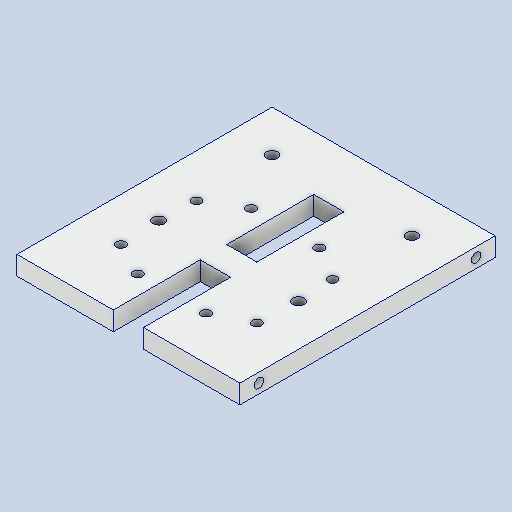
# Autodesk Inventor part: belt_liner_v2_Plate_4
Saved by Autodesk Inventor 2025.2 (Build 292293000, 293)
## iProperties
Created: 2025-01-05
Part Number: belt_liner_v2_Plate_4
Material: アルミニウム 6061
Document SubType Name: Modeling
Designer: haruy
Density: 2.7 g/cm^3
Appearance: アルミニウム - フラット
Author: haruy
Autodesk Inventor part; units mm, degrees
ref_plane "YZ Plane" through (0, 0, 0) normal (1, 0, 0) x (0, 1, 0)
ref_plane "XZ Plane" through (0, 0, 0) normal (0, 1, 0) x (-1, 0, 0)
derived "belt_liner_v2_Sketch_Base.ipt"
sketch "スケッチ4" plane through (0, 300, 0) normal (0, 1, 0) x (-1, 0, 0)
  line L0 (0, 0) -> (-15, 0) projected
  line L1 (-15, 0) -> (-15, -578.917) projected
  line L2 (-15, -578.917) -> (0, -578.917) projected
  line L3 (0, -578.917) -> (0, 0) projected
  line L4 (-4, -22.5) -> (-11, -22.5) projected
  line L5 (-11, -22.5) -> (-11, -0.5) projected
  line L6 (-11, -0.5) -> (-4, -0.5) projected
  line L7 (-4, -0.5) -> (-4, -22.5) projected
  line L8 (-4, -11.5) -> (-11, -11.5) projected
  line L9 (-4, -30.5) -> (-11, -30.5) projected
  line L10 (-11, -30.5) -> (-11, -52.5) projected
  line L11 (-11, -52.5) -> (-4, -52.5) projected
  line L12 (-4, -52.5) -> (-4, -30.5) projected
  line L13 (-4, -41.5) -> (-11, -41.5) projected
  line L14 (6.5, -7.5) -> (-21.5, -7.5) projected
  line L15 (-21.5, -7.5) -> (-21.5, -15.5) projected
  line L16 (-21.5, -15.5) -> (6.5, -15.5) projected
  line L17 (6.5, -15.5) -> (6.5, -7.5) projected
  line L18 (-11.5, -23) -> (-3.5, -23) projected
  line L19 (-3.5, -23) -> (-3.5, 0) projected
  line L20 (-3.5, 0) -> (-11.5, 0) projected
  line L21 (-11.5, 0) -> (-11.5, -23) projected
  circle A0 centre (1.5, -11.5) radius 4 projected
  circle A1 centre (-16.5, -11.5) radius 4 projected
  circle A2 centre (-26, -26.5) radius 11 projected
  circle A3 centre (-26, -26.5) radius 4 projected
  line L22 (-7.5, -52.5) -> (-7.5, 0) projected
  line L23 (0, -26.5) -> (-15, -26.5) projected
  circle A4 centre (11, -26.5) radius 11 projected
  circle A5 centre (11, -26.5) radius 4 projected
  circle A6 centre (1.5, -41.5) radius 4 projected
  line L24 (6.5, -37.5) -> (6.5, -45.5) projected
  line L25 (6.5, -45.5) -> (-21.5, -45.5) projected
  line L26 (-21.5, -45.5) -> (-21.5, -37.5) projected
  circle A7 centre (-16.5, -41.5) radius 4 projected
  line L27 (-21.5, -37.5) -> (6.5, -37.5) projected
  circle A8 centre (11, -56.5) radius 11 projected
  circle A9 centre (11, -56.5) radius 4 projected
  circle A10 centre (-26, -56.5) radius 11 projected
  circle A11 centre (-26, -56.5) radius 4 projected
  circle A12 centre (11, -56.5) radius 1.5 projected
  circle A13 centre (1.5, -41.5) radius 1.25 projected
  circle A14 centre (-16.5, -41.5) radius 1.25 projected
  circle A15 centre (-26, -56.5) radius 1.5 projected
  circle A16 centre (11, -26.5) radius 1.5 projected
  circle A17 centre (-26, -26.5) radius 1.5 projected
  circle A18 centre (1.5, -11.5) radius 1.25 projected
  circle A19 centre (-16.5, -11.5) radius 1.25 projected
  line L28 (22, 0) -> (-37, 0) projected
  line L29 (-37, 0) -> (-37, -67.5) projected
  line L30 (-37, -67.5) -> (22, -67.5) projected
  line L31 (22, -67.5) -> (22, 0) projected
  line L32 (-23, 0) -> (-28, 0) projected
  line L33 (-28, 0) -> (-28, -41) projected
  line L34 (-28, -41) -> (-23, -41) projected
  line L35 (-23, -41) -> (-23, 0) projected
  line L36 (-23, -10) -> (-28, -10) projected
  circle A20 centre (-25.5, -16) radius 1.25 projected
  circle A21 centre (-25.5, -16) radius 4 projected
  circle A22 centre (-25.5, -36) radius 4 projected
  circle A23 centre (-25.5, -36) radius 1.25 projected
  circle A24 centre (10.5, -36) radius 1.25 projected
  circle A25 centre (10.5, -16) radius 1.25 projected
  line L37 (-3.5, -53) -> (-11.5, -53)
  line L38 (-11.5, -53) -> (-11.5, -30)
  line L39 (-11.5, -30) -> (-3.5, -30)
  line L40 (-3.5, -30) -> (-3.5, -53)
  line L41 (2, 16.7328) -> (-17, 16.7328) projected
  line L42 (-17, 16.7328) -> (-17, 66.7328) projected
  line L43 (-17, 66.7328) -> (2, 66.7328) projected
  line L44 (2, 66.7328) -> (2, 16.7328) projected
  line L45 (-17, 61.7819) -> (-23, 61.7819) projected
  line L46 (-23, 61.7819) -> (-23, 36.7819) projected
  line L47 (-23, 36.7819) -> (-17, 36.7819) projected
  line L48 (-17, 36.7819) -> (-17, 61.7819) projected
  line L49 (18, 61.7819) -> (-33, 61.7819) projected
  line L50 (-33, 61.7819) -> (-33, 27.0059) projected
  line L51 (-33, 27.0059) -> (18, 27.0059) projected
  line L52 (18, 27.0059) -> (18, 61.7819) projected
  line L53 (-1.15, 66.7328) -> (-13.85, 66.7328) projected
  line L54 (-13.85, 66.7328) -> (-13.85, 140.5976) projected
  line L55 (-13.85, 140.5976) -> (-1.15, 140.5976) projected
  line L56 (-1.15, 140.5976) -> (-1.15, 66.7328) projected
  line L57 (7.85, 70.1693) -> (-22.85, 70.1693) projected
  line L58 (-22.85, 70.1693) -> (-22.85, 74.1693) projected
  line L59 (-22.85, 74.1693) -> (7.85, 74.1693) projected
  line L60 (7.85, 74.1693) -> (7.85, 70.1693) projected
  circle A26 centre (-17.85, 72.1693) radius 4 projected
  point P0 (-7.5, 0)
  point P1 (-7.5, 0)
  dimension "d1" = 0.5
  constraints: 8 end point, 3 other
  measures "d1" distance between parallel lines of L11 L37
extrude "押し出し1" add sketch "スケッチ4" against normal blind 5 contours L3 L14 L19 L0 | L28 L31 A4 A25 L3 L16 L17 L14 | L14 A0 L3 | L3 A0 L16 L19 L14 | A0 L3 | L3 A0 | L14 L17 L16 A0 | L31 A8 L3 L25 L24 L27 A4 | A4 A25 | L21 L14 L1 L0 | L16 L3 L23 L22 L18 L19 | A0 L16 L3 | L3 L27 L40 L39 L22 L23 | A25 A4 | A4 A25 | A8 | L31 L30 A8 | L1 L14 L15 L16 A2 A21 L35 L28 | L21 L16 L1 A1 L14 | L27 A6 L3 | L3 A6 L25 L40 L27 | L23 L1 L16 L21 L18 L22 | L22 L39 L38 L27 L1 L23 | A8 L30 L3 | L3 L30 L1 L25 L38 L37 L40 | L1 A1 L14 | L35 L36 L33 L28 | A6 L3 | L3 A6 | L27 L24 L25 A6 | A2 A22 L35 A3 A21 | L1 L27 L26 L25 A10 L29 A2 A22 L33 L34 L35 | L3 A6 L25 | A1 L1 | L1 A1 | A1 L16 L15 L14 | L33 A21 A2 L29 L28 | L35 A21 L33 L36 | L16 A1 L1 | L27 L38 L25 L1 A7 | L1 A7 L27 | A21 L35 A2 | A2 L35 A21 | A22 L35 A2 | A2 L35 A22 | L30 A10 L1 | L35 A2 A20 L33 A21 | A7 L1 | L1 A7 | A7 L25 L26 L27 | L35 A21 L33 A2 A20 | L35 A3 L33 A21 | L35 A22 L33 A2 | A2 L33 A22 L35 | L35 L34 L33 A22 | A10 | L30 L29 A10 | A2 A21 L33 A3 A22 | L33 A2 A21 | L1 L25 A7 | A20 A2 | A2 A20 | L35 A3 L33 | A3 L35 | A21 A2 L33 | L33 A22 A2 | A2 A22 L33 | A22 L33 A3 L35 | L33 A3 | A5 | A9 | A11 | A23 | A24
extrude "押し出し2" cut sketch "スケッチ4" against normal blind 5 contours A25 A4 | A4 A25 | A20 A2 | A2 A20 | A23 | A24 picked at (10.5247, -16.0944) picked at (10.4649, -15.2634)
ref_plane "作業平面1" through (7.5, 300, 0) normal (1, 0, 0) x (0, 0, -1)
sketch "スケッチ2" plane through (37, 300, 0) normal (1, 0, 0) x (0, 0, -1)
  line L0 (0, 0) -> (0, -5) projected
  line L1 (0, 0) -> (67.5, 0) projected
  line L2 (67.5, 0) -> (67.5, -5) projected
  line L3 (67.5, -5) -> (0, -5) projected
  point P0 (0, -300)
  point P1 (5, -2.5)
  point P2 (62.5, -2.5)
  dimension "d7" = 5
  dimension "d8" = 2.5
  dimension "d9" = 5
  dimension "d10" = 2.5
  measures "d7" distance from line of L0 point (5, -2.5)
  measures "d8" distance from line of point (5, -2.5) L1
  measures "d9" distance from line of point (62.5, -2.5) L2
  measures "d10" distance from line of point (62.5, -2.5) L3
hole "穴1" at (37, 297.5, -5) at (37, 297.5, -62.5) direction (-1, 0, 0) diameter 2.5 depth 5 tip angle 118
mirror "ミラー1" about plane through (7.5, 300, 0) normal (1, 0, 0) of "穴1"
equation "\"d9\" = d7"
equation "\"d10\" = d8"
